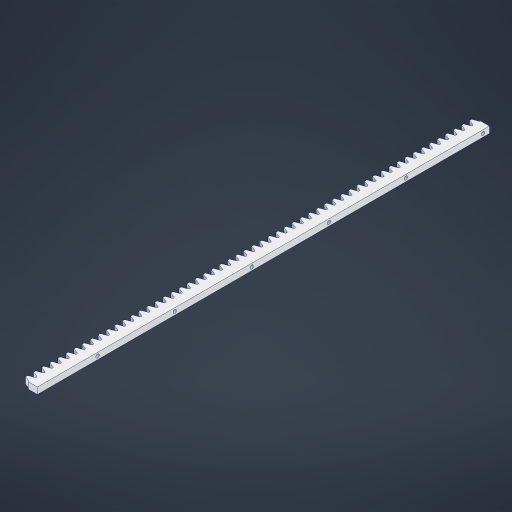
# Autodesk Inventor part: CLIM_001_ClimbRack
Saved by Autodesk Inventor 2024.2 (Build 282272000, 272)
## iProperties
Created: 2024-08-07
Part Number: CLIM_001_ClimbRack
Material: Aluminum 6061
Document SubType Name: Modeling
Designer: Bryan
Density: 2.7 g/cm^3
Appearance: Aluminum - Flat
Mass: 90.807 g
Surface Area: 195.243 cm^2
Volume: 33.6322 cm^3
Author: Bryan
Autodesk Inventor part; units mm, degrees
ref_plane "YZ Plane" through (0, 0, 0) normal (1, 0, 0) x (0, 1, 0)
ref_plane "XZ Plane" through (0, 0, 0) normal (0, 1, 0) x (-1, 0, 0)
ref_plane "XY Plane" through (0, 0, 0) normal (0, 0, 1) x (1, 0, 0)
sketch "Sketch4" plane through (0, 0, 0) normal (0, 1, 0) x (-1, 0, 0)
  line L0 (0, 0) -> (-8.89, 0)
  line L1 (-8.89, 0) -> (-8.89, -446.8601)
  line L2 (-8.89, -446.8601) -> (0, -446.8601)
  line L3 (0, -446.8601) -> (0, 0)
  line L4 (3.175, 0) -> (3.175, -446.8601) construction
  line L5 (5.715, 0) -> (5.715, -446.8601) construction
  line L6 (5.715, -2.9194) -> (5.715, -5.0602)
  line L7 (5.715, -5.0602) -> (0, -7.1403)
  line L8 (5.715, -2.9194) -> (0, -0.8393)
  point P0 (-4.445, -446.8601)
  point P1 (3.175, -1.9949)
  point P2 (3.175, -5.9847)
  point P3 (5.715, -3.9898)
  dimension "d23" = 8.89
  dimension "d24" = 446.8601
  dimension "d25" = 3.175
  dimension "d26" = 2.54
  dimension "d29" = 3.9898
  dimension "d31" = 70
  dimension "d32" = 3.9898
  constraints: 18 end point, 8 point on line, 4 horizontal alignment, 2 midpoint, 2 parallel, 2 vertical, 1 equal length, 1 horizontal, 1 perpendicular
  measures "d23" distance of L2.end L1.end
  measures "d24" distance of L1.end L0.end
  measures "d25" distance between parallel lines of L3 L4
  measures "d26" distance between parallel lines of L4 L5
  measures "d29" distance of point (3.175, -1.995) point (3.175, -5.985)
  measures "d31" angle of L3 L7
  measures "d32" distance from line of point (5.715, -3.99) L0
extrude "Extrusion3" add sketch "Sketch4" against normal blind 6.35 contours L3 L2 L1 L0
extrude "Extrusion4" add sketch "Sketch4" against normal blind 6.35 contours L8 L6 L7 L3
fillet "Fillet1" radius 0.9652 2 edges at (0, -3.175, -0.8393) (0, -3.175, -7.1403)
pattern_linear "Rectangular Pattern1" count 56 spacing 7.9796 along (0, 0, -1) of "Fillet1", "Extrusion4"
sketch "Sketch5" plane through (8.89, 0, 0) normal (1, 0, 0) x (0, 0, -1)
  line L0 (0, 0) -> (446.8601, 0) projected
  line L1 (0, 0) -> (0, -6.35) projected
  line L2 (446.8601, -6.35) -> (0, -6.35) projected
  line L3 (446.8601, 0) -> (446.8601, -6.35) projected
  circle A0 centre (-16.6899, -3.175) radius 1.7272
  circle A1 centre (59.5101, -3.175) radius 1.7272
  circle A2 centre (135.7101, -3.175) radius 1.7272
  circle A3 centre (211.9101, -3.175) radius 1.7272
  circle A4 centre (288.1101, -3.175) radius 1.7272
  circle A5 centre (364.3101, -3.175) radius 1.7272
  circle A6 centre (440.5101, -3.175) radius 1.7272
  point P0 (0, -3.175)
  dimension "d41" = 446.8601
  dimension "d42" = 3.4544
  dimension "d46" = 76.2
  dimension "d65" = 6.35
  constraints: 7 centre point, 1 horizontal, 1 horizontal alignment, 1 midpoint, 12 other
  measures "d41" distance of L2.start L1.end
  measures "d42" diameter of A0
  measures "d46" distance of A0.centre A1.centre
  measures "d65" distance from line of L3 A6.centre
extrude "Extrusion5" cut sketch "Sketch5" against normal blind 6.35 contours A0 | A1 | A2 | A3 | A4 | A5 | A6
thread "Thread1" size "8-32 UNC" class "2B" standard "ANSI Unified Screw Threads" full length
thread "Thread2" size "8-32 UNC" class "2B" standard "ANSI Unified Screw Threads" full length
thread "Thread3" size "8-32 UNC" class "2B" standard "ANSI Unified Screw Threads" full length
thread "Thread4" size "8-32 UNC" class "2B" standard "ANSI Unified Screw Threads" full length
thread "Thread5" size "8-32 UNC" class "2B" standard "ANSI Unified Screw Threads" full length
thread "Thread6" size "8-32 UNC" class "2B" standard "ANSI Unified Screw Threads" full length
equation "\"d24\" = length"
equation "\"d25\" = 1.25 * mod"
equation "\"d26\" = mod"
equation "\"d29\" = 1.5708 * mod"
equation "\"d32\" = 1.5708 * mod"
equation "\"d35\" = 0.38 * mod"
equation "\"d40\" = 3.14159 * mod"
equation "\"a\" = 20deg"
equation "\"length\" = 446.860139"
equation "\"mod\" = 2.54"
body "Solid2"
